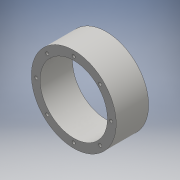
# Autodesk Inventor part: sprocketsHolder
Saved by Autodesk Inventor 2016 (Build 200138000, 138)
## iProperties
Created: 2016-05-15
Part Number: sprocketsHolder
Material: Generic
Document SubType Name: Modeling
Designer: Henrik Samuelsson
Density: 1 g/cm^3
Appearance: Default
Author: Henrik Samuelsson
Autodesk Inventor part; units mm, degrees
ref_plane "YZ Plane" through (0, 0, 0) normal (1, 0, 0) x (0, 1, 0)
ref_plane "XZ Plane" through (0, 0, 0) normal (0, 1, 0) x (-1, 0, 0)
ref_plane "XY Plane" through (0, 0, 0) normal (0, 0, 1) x (1, 0, 0)
sketch "Sketch1" plane through (0, 0, 0) normal (0, 1, 0) x (-1, 0, 0)
  circle A0 centre (0, 0) radius 34
  circle A1 centre (9.5, 0) radius 1.6
  circle A2 centre (4.75, 8.2272) radius 1.6
  circle A3 centre (-4.75, 8.2272) radius 1.6
  circle A4 centre (-9.5, 0) radius 1.6
  circle A5 centre (-4.75, -8.2272) radius 1.6
  circle A6 centre (4.75, -8.2272) radius 1.6
  circle A7 centre (30, 0) radius 1.225
  circle A8 centre (21.2132, 21.2132) radius 1.225
  circle A9 centre (0, 30) radius 1.225
  circle A10 centre (-21.2132, 21.2132) radius 1.225
  circle A11 centre (-30, 0) radius 1.225
  circle A12 centre (-21.2132, -21.2132) radius 1.225
  circle A13 centre (0, -30) radius 1.225
  circle A14 centre (21.2132, -21.2132) radius 1.225
  dimension "d0" = 68
  dimension "d1" = 3.2
  dimension "d2" = 9.5
  dimension "d3" = 0
  dimension "d6" = 360
  dimension "d10" = 2.45
  dimension "d11" = 0
  dimension "d12" = 30
  dimension "d15" = 360
  constraints: 15 centre point, 1 coincident, 30 other
  measures "d0" diameter of A0
  measures "d1" diameter of A1
  measures "d2" distance of A1.centre point (0, 0)
  measures "d3" vertical distance of point (0, 0) A1.centre
  measures "d10" diameter of A7
  measures "d11" vertical distance of point (0, 0) A7.centre
  measures "d12" distance of point (0, 0) A7.centre
extrude "Extrusion3" add sketch "Sketch1" along normal blind 5
sketch "Sketch5" plane through (0, 0, 0) normal (0, -1, 0) x (1, 0, 0)
  circle A0 centre (0, 0) radius 34 projected
  circle A1 centre (21.2132, 21.2132) radius 1.225 projected
  circle A2 centre (30, 0) radius 1.225 projected
  circle A3 centre (21.2132, -21.2132) radius 1.225 projected
  circle A4 centre (0, -30) radius 1.225 projected
  circle A5 centre (-21.2132, -21.2132) radius 1.225 projected
  circle A6 centre (-30, 0) radius 1.225 projected
  circle A7 centre (-21.2132, 21.2132) radius 1.225 projected
  circle A8 centre (0, 30) radius 1.225 projected
  circle A9 centre (0, 0) radius 27
  circle A10 centre (21.2132, 21.2132) radius 1.225
  circle A11 centre (30, 0) radius 1.225
  circle A12 centre (21.2132, -21.2132) radius 1.225
  circle A13 centre (0, -30) radius 1.225
  circle A14 centre (-21.2132, -21.2132) radius 1.225
  circle A15 centre (-30, 0) radius 1.225
  circle A16 centre (-21.2132, 21.2132) radius 1.225
  circle A17 centre (0, 30) radius 1.225 projected
  circle A18 centre (0, 30) radius 1.225
  circle A19 centre (0, 0) radius 34
  dimension "d21" = 54
  constraints: 10 centre point, 10 coincident, 8 concentric
  measures "d21" diameter of A9
extrude "Extrusion4" add sketch "Sketch5" along normal blind 26
sketch "Sketch6" plane through (0, 5, 0) normal (0, 1, 0) x (1, 0, 0)
  circle A0 centre (0, 0) radius 34
  constraints: 1 centre point, 1 coincident
extrude "Extrusion5" cut sketch "Sketch6" against normal blind 5
body "Solid3"
